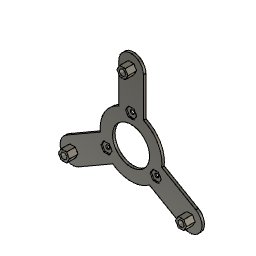
Limitswitch_steering_holder_base (Autodesk Fusion 360 archive; units mm, degrees)
design "front_speed_sensor"
Autodesk Fusion 360 part; units mm, degrees
sketch "Sketch1" plane through (0, 0, 0) normal (0, 1, 0) x (1, 0, 0)
  circle A0 centre (0, 0) radius 15
  circle A1 centre (0, 0) radius 25
  line L0 (0, 0) -> (0, -54.75) construction
  circle A2 centre (0, -54.75) radius 2.435
  line L1 (4.5611, -54.75) -> (2.2805, -50.8)
  line L2 (2.2805, -50.8) -> (-2.2805, -50.8)
  line L3 (-2.2805, -50.8) -> (-4.5611, -54.75)
  line L4 (-4.5611, -54.75) -> (-2.2805, -58.7)
  line L5 (-2.2805, -58.7) -> (2.2805, -58.7)
  line L6 (2.2805, -58.7) -> (4.5611, -54.75)
  line L7 (-10, -22.9129) -> (-10, -54.75)
  arc A3 (-10, -54.75) -> (10, -54.75) centre (0, -54.75) ccw
  line L8 (10, -54.75) -> (10, -22.9129)
  line L9 (0, 0) -> (47.4149, 27.375) construction
  line L10 (45.1344, 31.325) -> (42.8538, 27.375)
  circle A4 centre (47.4149, 27.375) radius 2.435
  line L11 (51.976, 27.375) -> (49.6954, 31.325)
  line L12 (42.8538, 27.375) -> (45.1344, 23.425)
  line L13 (49.6954, 23.425) -> (51.976, 27.375)
  line L14 (45.1344, 23.425) -> (49.6954, 23.425)
  arc A5 (52.4149, 18.7147) -> (42.4149, 36.0353) centre (47.4149, 27.375) ccw
  line L15 (49.6954, 31.325) -> (45.1344, 31.325)
  line L16 (42.4149, 36.0353) -> (14.8431, 20.1167)
  line L17 (24.8431, 2.7962) -> (52.4149, 18.7147)
  line L18 (0, 0) -> (-47.4149, 27.375) construction
  line L19 (-49.6954, 23.425) -> (-45.1344, 23.425)
  circle A6 centre (-47.4149, 27.375) radius 2.435
  line L20 (-49.6954, 31.325) -> (-51.976, 27.375)
  line L21 (-45.1344, 23.425) -> (-42.8538, 27.375)
  line L22 (-45.1344, 31.325) -> (-49.6954, 31.325)
  line L23 (-42.8538, 27.375) -> (-45.1344, 31.325)
  arc A7 (-42.4149, 36.0353) -> (-52.4149, 18.7147) centre (-47.4149, 27.375) ccw
  line L24 (-51.976, 27.375) -> (-49.6954, 23.425)
  line L25 (-52.4149, 18.7147) -> (-24.8431, 2.7962)
  line L26 (-14.8431, 20.1167) -> (-42.4149, 36.0353)
  point P0 (0, -54.75)
  point P1 (47.4149, 27.375)
  point P2 (-47.4149, 27.375)
  dimension "d1" = 30
  dimension "d2" = 50
  dimension "d3" = 7.9
  dimension "d4" = 4.87
  dimension "d5" = 50.8
  dimension "d6" = 10
  dimension "d8" = 360
  constraint coincident A0.centre A1.centre
  constraint concentric A0 A1
  constraint vertical L0
  constraint coincident P0 L0.end
  constraint horizontal L2
  constraint coincident A1 L7.start
  constraint vertical L7
  constraint tangent L7 A3
  constraint coincident A1 L8.end
  constraint parallel L7 L8
  constraint horizontal L7.end A3.end
  constraint vertical A0.centre L0.end
  measures "d1" diameter of A0
  measures "d2" diameter of A1
  measures "d3" distance of L2 L5
  measures "d4" diameter of A2
  measures "d5" distance of A0.centre L2
  measures "d6" radius of A3
extrude "Extrude1" add sketch "Sketch1" along normal blind 2 contours A1 | A1 A5 L16 L17 | A1 L7 A3 L8 | A1 A7 L25 L26 | L1 L2 L3 L4 L5 L6 | L10 L11 L12 L13 L14 L15 | L19 L20 L21 L22 L23 L24
sketch "Sketch2" plane through (0, 0, 0) normal (0, -1, 0) x (1, 0, 0)
  circle A0 centre (0, 0) radius 15
  circle A1 centre (47.4149, -27.375) radius 2.435
  circle A2 centre (0, 54.75) radius 2.435
  circle A3 centre (-47.4149, -27.375) radius 2.435
  line L0 (-42.4149, -36.0353) -> (-14.8431, -20.1167)
  arc A4 (-14.8431, -20.1167) -> (14.8431, -20.1167) centre (0, 0) ccw
  line L1 (14.8431, -20.1167) -> (42.4149, -36.0353)
  arc A5 (42.4149, -36.0353) -> (52.4149, -18.7147) centre (47.4149, -27.375) ccw
  line L2 (52.4149, -18.7147) -> (24.8431, -2.7962)
  arc A6 (24.8431, -2.7962) -> (10, 22.9129) centre (0, 0) ccw
  line L3 (10, 22.9129) -> (10, 54.75)
  arc A7 (10, 54.75) -> (-10, 54.75) centre (0, 54.75) ccw
  line L4 (-10, 54.75) -> (-10, 22.9129)
  arc A8 (-10, 22.9129) -> (-24.8431, -2.7962) centre (0, 0) ccw
  line L5 (-24.8431, -2.7962) -> (-52.4149, -18.7147)
  arc A9 (-52.4149, -18.7147) -> (-42.4149, -36.0353) centre (-47.4149, -27.375) ccw
  line L6 (2.2372, 50.875) -> (4.4745, 54.75)
  line L7 (4.4745, 54.75) -> (2.2372, 58.625)
  line L8 (2.2372, 58.625) -> (-2.2372, 58.625)
  line L9 (-2.2372, 58.625) -> (-4.4745, 54.75)
  line L10 (-4.4745, 54.75) -> (-2.2372, 50.875)
  line L11 (-2.2372, 50.875) -> (2.2372, 50.875)
  line L12 (-51.8894, -27.375) -> (-49.6521, -31.25)
  line L13 (-45.1777, -23.5) -> (-49.6521, -23.5)
  line L14 (-42.9404, -27.375) -> (-45.1777, -23.5)
  line L15 (-49.6521, -31.25) -> (-45.1777, -31.25)
  circle A10 centre (-47.4149, -27.375) radius 2.435
  line L16 (-45.1777, -31.25) -> (-42.9404, -27.375)
  line L17 (-49.6521, -23.5) -> (-51.8894, -27.375)
  line L18 (49.6521, -31.25) -> (51.8894, -27.375)
  line L19 (42.9404, -27.375) -> (45.1777, -31.25)
  line L20 (45.1777, -23.5) -> (42.9404, -27.375)
  line L21 (51.8894, -27.375) -> (49.6521, -23.5)
  circle A11 centre (47.4149, -27.375) radius 2.435
  line L22 (49.6521, -23.5) -> (45.1777, -23.5)
  line L23 (45.1777, -31.25) -> (49.6521, -31.25)
  point P0 (0, 54.75)
  point P1 (-47.4149, -27.375)
  point P2 (47.4149, -27.375)
  dimension "d11" = 7.75
  dimension "d13" = 360
  constraint coincident P0 A2.centre
  constraint horizontal L11
  measures "d11" distance of L8 L11
extrude "Extrude2" add sketch "Sketch2" along normal blind 7 contours L6 L7 L8 L9 L10 L11 | L12 L13 L14 L15 L16 L17 | L18 L19 L20 L21 L22 L23
sketch "Sketch3" plane through (0, 2, 0) normal (0, 1, 0) x (-1, 0, 0)
  circle A0 centre (0, 0) radius 15
  circle A1 centre (-47.4149, -27.375) radius 2.435
  circle A2 centre (0, 54.75) radius 2.435
  circle A3 centre (47.4149, -27.375) radius 2.435
  line L0 (14.8431, -20.1167) -> (42.4149, -36.0353)
  arc A4 (42.4149, -36.0353) -> (52.4149, -18.7147) centre (47.4149, -27.375) ccw
  line L1 (52.4149, -18.7147) -> (24.8431, -2.7962)
  arc A5 (24.8431, -2.7962) -> (10, 22.9129) centre (0, 0) ccw
  line L2 (10, 22.9129) -> (10, 54.75)
  arc A6 (10, 54.75) -> (-10, 54.75) centre (0, 54.75) ccw
  line L3 (-10, 54.75) -> (-10, 22.9129)
  arc A7 (-10, 22.9129) -> (-24.8431, -2.7962) centre (0, 0) ccw
  line L4 (-24.8431, -2.7962) -> (-52.4149, -18.7147)
  arc A8 (-52.4149, -18.7147) -> (-42.4149, -36.0353) centre (-47.4149, -27.375) ccw
  line L5 (-42.4149, -36.0353) -> (-14.8431, -20.1167)
  arc A9 (-14.8431, -20.1167) -> (14.8431, -20.1167) centre (0, 0) ccw
  line L6 (0, 54.75) -> (0, 15) construction
  circle A10 centre (0, 23) radius 3
  circle A11 centre (0, 23) radius 1.575
  circle A12 centre (-19.9186, -11.5) radius 3
  circle A13 centre (-19.9186, -11.5) radius 1.575
  circle A14 centre (19.9186, -11.5) radius 3
  circle A15 centre (19.9186, -11.5) radius 1.575
  dimension "d16" = 8
  dimension "d17" = 6
  dimension "d18" = 3.15
  dimension "d20" = 360
  constraint coincident A2.centre A6.centre
  constraint coincident A0 L6.end
  constraint vertical L6
  constraint coincident L6 A10.centre
  constraint concentric A10 A11
  measures "d16" distance of L6.end A10.centre
  measures "d17" diameter of A10
  measures "d18" diameter of A11
extrude "Extrude6" cut sketch "Sketch3" against normal up to surface (2 mm away) contours A11 | A13 | A15
sketch "Sketch5" plane through (0, 0, 0) normal (0, -1, 0) x (1, 0, 0)
  circle A0 centre (19.9186, -11.5) radius 1.575
  circle A1 centre (0, 23) radius 1.575
  circle A2 centre (-19.9186, -11.5) radius 1.575
  line L0 (-2.2372, 50.875) -> (-4.4745, 54.75)
  line L1 (-4.4745, 54.75) -> (-2.2372, 58.625)
  line L2 (-2.2372, 58.625) -> (2.2372, 58.625)
  line L3 (2.2372, 58.625) -> (4.4745, 54.75)
  line L4 (4.4745, 54.75) -> (2.2372, 50.875)
  line L5 (2.2372, 50.875) -> (-2.2372, 50.875)
  line L6 (-49.6521, -23.5) -> (-45.1777, -23.5)
  line L7 (-45.1777, -23.5) -> (-42.9404, -27.375)
  line L8 (-42.9404, -27.375) -> (-45.1777, -31.25)
  line L9 (-45.1777, -31.25) -> (-49.6521, -31.25)
  line L10 (-49.6521, -31.25) -> (-51.8894, -27.375)
  line L11 (-51.8894, -27.375) -> (-49.6521, -23.5)
  line L12 (45.1777, -31.25) -> (42.9404, -27.375)
  line L13 (42.9404, -27.375) -> (45.1777, -23.5)
  line L14 (45.1777, -23.5) -> (49.6521, -23.5)
  line L15 (49.6521, -23.5) -> (51.8894, -27.375)
  line L16 (51.8894, -27.375) -> (49.6521, -31.25)
  line L17 (49.6521, -31.25) -> (45.1777, -31.25)
  circle A3 centre (0, 0) radius 15
  line L18 (-42.4149, -36.0353) -> (-14.8431, -20.1167)
  arc A4 (-14.8431, -20.1167) -> (14.8431, -20.1167) centre (0, 0) ccw
  line L19 (14.8431, -20.1167) -> (42.4149, -36.0353)
  arc A5 (42.4149, -36.0353) -> (52.4149, -18.7147) centre (47.4149, -27.375) ccw
  line L20 (52.4149, -18.7147) -> (24.8431, -2.7962)
  arc A6 (24.8431, -2.7962) -> (10, 22.9129) centre (0, 0) ccw
  line L21 (10, 22.9129) -> (10, 54.75)
  arc A7 (10, 54.75) -> (-10, 54.75) centre (0, 54.75) ccw
  line L22 (-10, 54.75) -> (-10, 22.9129)
  arc A8 (-10, 22.9129) -> (-24.8431, -2.7962) centre (0, 0) ccw
  line L23 (-24.8431, -2.7962) -> (-52.4149, -18.7147)
  arc A9 (-52.4149, -18.7147) -> (-42.4149, -36.0353) centre (-47.4149, -27.375) ccw
  line L24 (2.2372, 26.875) -> (-2.2372, 26.875)
  line L25 (-2.2372, 26.875) -> (-4.4745, 23)
  line L26 (-4.4745, 23) -> (-2.2372, 19.125)
  line L27 (-2.2372, 19.125) -> (2.2372, 19.125)
  line L28 (2.2372, 19.125) -> (4.4745, 23)
  line L29 (4.4745, 23) -> (2.2372, 26.875)
  line L30 (-22.1558, -15.375) -> (-17.6814, -15.375)
  line L31 (-22.1558, -7.625) -> (-24.393, -11.5)
  circle A10 centre (-19.9186, -11.5) radius 1.575
  line L32 (-17.6814, -15.375) -> (-15.4441, -11.5)
  line L33 (-24.393, -11.5) -> (-22.1558, -15.375)
  line L34 (-15.4441, -11.5) -> (-17.6814, -7.625)
  line L35 (-17.6814, -7.625) -> (-22.1558, -7.625)
  line L36 (24.393, -11.5) -> (22.1558, -7.625)
  line L37 (17.6814, -15.375) -> (22.1558, -15.375)
  circle A11 centre (19.9186, -11.5) radius 1.575
  line L38 (22.1558, -7.625) -> (17.6814, -7.625)
  line L39 (22.1558, -15.375) -> (24.393, -11.5)
  line L40 (17.6814, -7.625) -> (15.4441, -11.5)
  line L41 (15.4441, -11.5) -> (17.6814, -15.375)
  point P0 (0, 23)
  point P1 (-19.9186, -11.5)
  point P2 (19.9186, -11.5)
  dimension "d32" = 7.75
  dimension "d34" = 360
  constraint coincident P0 A1.centre
  constraint horizontal L27
  measures "d32" distance of L24 L27
extrude "Extrude7" cut sketch "Sketch5" against normal up to surface (1 mm away) contours L24 L25 L26 L27 L28 L29 | L30 L31 L32 L33 L34 L35 | L36 L37 L38 L39 L40 L41
